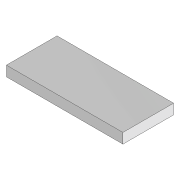
# Autodesk Inventor part: Bottom
Saved by Autodesk Inventor 2022.5 (Build 265521000, 521)
## iProperties
Created: 2020-02-29
Part Number: Bottom
Document SubType Name: Modeling
Designer: Administrator
Density: 1 g/cm^3
Material: Generic
Appearance: White
Author: Administrator
Autodesk Inventor part; units mm, degrees
ref_plane "YZ Plane" through (0, 0, 0) normal (1, 0, 0) x (0, 1, 0)
ref_plane "XZ Plane" through (0, 0, 0) normal (0, 1, 0) x (-1, 0, 0)
ref_plane "XY Plane" through (0, 0, 0) normal (0, 0, 1) x (1, 0, 0)
sketch "Sketch1" plane through (0, 0, 0) normal (0, 0, 1) x (1, 0, 0)
  line L0 (0, 0) -> (46, 0)
  line L1 (46, 0) -> (46, 20)
  line L2 (46, 20) -> (0, 20)
  line L3 (0, 20) -> (0, 0)
  line L4 (0, 0) -> (-46, 0)
  line L5 (-46, 0) -> (-46, -20)
  line L6 (-46, -20) -> (0, -20)
  line L7 (0, -20) -> (0, 0)
  line L8 (-46, -20) -> (46, -20)
  line L9 (46, -20) -> (46, 20)
  line L10 (46, 20) -> (-46, 20)
  line L11 (-46, 20) -> (-46, -20)
  point P0 (0, 20)
  point P1 (0, -20)
  dimension "d7" = 40
  dimension "d8" = 92
  constraints: 24 end point, 6 parallel, 3 horizontal, 3 perpendicular, 2 collinear
  measures "d7" distance of L8.end L1.end
  measures "d8" distance of L1.end L10.end
extrude "Extrusion1" add sketch "Sketch1" along normal blind 8
sketch "Sketch2" plane through (0, 0, 0) normal (0, 0, -1) x (-1, 0, 0)
  circle A0 centre (24, 16) radius 1.25 construction
  circle A1 centre (-33, 16.5) radius 1.5
  circle A2 centre (-14, 16) radius 1.25 construction
  circle A3 centre (14, 16) radius 1.25 construction
  circle A4 centre (4.5, 16.5) radius 1.5
  circle A5 centre (-5, -16.5) radius 1.5
  circle A6 centre (32.5, -16.5) radius 1.5
  point P0 (0, 0)
extrude "Extrusion2" cut sketch "Sketch2" against normal through all
body "Solid1"
